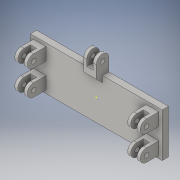
# Autodesk Inventor part: wheel mount
Saved by Autodesk Inventor 2016 (Build 200138000, 138)
## iProperties
Created: 2017-06-27
Part Number: wheel mount
Material: Generic
Document SubType Name: Modeling
Designer: andon
Density: 1 g/cm^3
Appearance: Default
Author: andon
Autodesk Inventor part; units mm, degrees
ref_plane "YZ Plane" through (0, 0, 0) normal (1, 0, 0) x (0, 1, 0)
ref_plane "XZ Plane" through (0, 0, 0) normal (0, 1, 0) x (-1, 0, 0)
ref_plane "XY Plane" through (0, 0, 0) normal (0, 0, 1) x (1, 0, 0)
sketch "Sketch1" plane through (0, 0, 0) normal (0, 0, 1) x (1, 0, 0)
  line L0 (-266.7, 88.9) -> (266.7, 88.9)
  line L1 (266.7, 88.9) -> (266.7, -88.9)
  line L2 (266.7, -88.9) -> (-266.7, -88.9)
  line L3 (-266.7, -88.9) -> (-266.7, 88.9)
  line L4 (-266.7, 88.9) -> (266.7, -88.9) construction
  line L5 (266.7, 88.9) -> (-266.7, -88.9) construction
  point P0 (0, 0)
  dimension "d0" = 533.4
  dimension "d1" = 177.8
  constraints: 12 end point, 2 midpoint, 2 parallel, 1 horizontal, 1 perpendicular
  measures "d0" distance of L1.end L2.end
  measures "d1" distance of L0.end L1.end
extrude "Extrusion1" add sketch "Sketch1" along normal blind 25.4
sketch "Sketch2" plane through (0, 0, 25.4) normal (0, 0, 1) x (1, 0, 0)
  line L0 (-254, -76.2) -> (254, -76.2)
  line L1 (254, -76.2) -> (254, 76.2)
  line L2 (254, 76.2) -> (-254, 76.2)
  line L3 (-254, 76.2) -> (-254, -76.2)
  line L4 (-254, -76.2) -> (254, 76.2) construction
  line L5 (254, -76.2) -> (-254, 76.2) construction
  line L6 (-254, 76.2) -> (-203.2, 76.2)
  line L7 (-203.2, 76.2) -> (-203.2, 25.4)
  line L8 (-203.2, 25.4) -> (-254, 25.4)
  line L9 (-254, 25.4) -> (-254, 76.2)
  line L10 (-254, -76.2) -> (-203.2, -76.2)
  line L11 (-203.2, -76.2) -> (-203.2, -25.4)
  line L12 (-203.2, -25.4) -> (-254, -25.4)
  line L13 (-254, -25.4) -> (-254, -76.2)
  line L14 (254, 76.2) -> (203.2, 76.2)
  line L15 (203.2, 76.2) -> (203.2, 25.4)
  line L16 (203.2, 25.4) -> (254, 25.4)
  line L17 (254, 25.4) -> (254, 76.2)
  line L18 (254, -76.2) -> (203.2, -76.2)
  line L19 (203.2, -76.2) -> (203.2, -25.4)
  line L20 (203.2, -25.4) -> (254, -25.4)
  line L21 (254, -25.4) -> (254, -76.2)
  point P0 (0, 0)
  dimension "d4" = 508
  dimension "d5" = 152.4
  dimension "d6" = 50.8
  dimension "d7" = 50.8
  dimension "d8" = 50.8
  dimension "d9" = 50.8
  dimension "d10" = 50.8
  dimension "d11" = 50.8
  dimension "d12" = 50.8
  dimension "d13" = 50.8
  constraints: 44 end point, 10 parallel, 5 horizontal, 5 perpendicular, 2 midpoint
  measures "d4" distance of L2.end L1.end
  measures "d5" distance of L1.end L0.end
  measures "d6" distance of L7.end L8.end
  measures "d7" distance of L6.end L7.end
  measures "d8" distance of L12.end L11.end
  measures "d9" distance of L11.end L10.end
  measures "d10" distance of L16.end L15.end
  measures "d11" distance of L15.end L14.end
  measures "d12" distance of L19.end L20.end
  measures "d13" distance of L18.end L19.end
extrude "Extrusion2" add sketch "Sketch2" along normal blind 76.2 contours L3 L12 L11 L0 | L19 L20 L1 L0 | L3 L2 L7 L8 | L16 L15 L2 L1
sketch "Sketch3" plane through (0, 0, 101.6) normal (0, 0, 1) x (1, 0, 0)
  line L0 (-254, 76.2) -> (-203.2, 76.2) projected
  line L1 (-203.2, 25.4) -> (-254, 25.4) projected
  line L2 (-241.3, 76.2) -> (-215.9, 76.2)
  line L3 (-215.9, 76.2) -> (-215.9, 25.4)
  line L4 (-215.9, 25.4) -> (-241.3, 25.4)
  line L5 (-241.3, 25.4) -> (-241.3, 76.2)
  line L6 (-254, -25.4) -> (-203.2, -25.4) projected
  line L7 (-254, -76.2) -> (-203.2, -76.2) projected
  line L8 (-241.3, -25.4) -> (-215.9, -25.4)
  line L9 (-215.9, -25.4) -> (-215.9, -76.2)
  line L10 (-215.9, -76.2) -> (-241.3, -76.2)
  line L11 (-241.3, -76.2) -> (-241.3, -25.4)
  line L12 (254, -25.4) -> (203.2, -25.4) projected
  line L13 (203.2, -76.2) -> (254, -76.2) projected
  line L14 (215.9, -25.4) -> (241.3, -25.4)
  line L15 (241.3, -25.4) -> (241.3, -76.2)
  line L16 (241.3, -76.2) -> (215.9, -76.2)
  line L17 (215.9, -76.2) -> (215.9, -25.4)
  line L18 (254, 76.2) -> (203.2, 76.2) projected
  line L19 (241.3, 25.4) -> (215.9, 25.4)
  line L20 (215.9, 25.4) -> (215.9, 76.2)
  line L21 (215.9, 76.2) -> (241.3, 76.2)
  line L22 (241.3, 76.2) -> (241.3, 25.4)
  point P0 (0, 0)
  constraints: 32 end point, 9 point on line, 8 parallel, 4 horizontal, 4 perpendicular
extrude "Extrusion3" cut sketch "Sketch3" against normal blind 50.8
fillet "Fillet1" radius 25.4 16 edges at (-247.65, 76.2, 101.6) (-209.55, 76.2, 101.6) (-209.55, 25.4, 101.6) (-247.65, 25.4, 101.6) (-247.65, -25.4, 101.6) (-247.65, -76.2, 101.6) (-209.55, -25.4, 101.6) (-209.55, -76.2, 101.6) (247.65, 76.2, 101.6) (209.55, 76.2, 101.6) (209.55, 25.4, 101.6) (247.65, 25.4, 101.6) (247.65, -25.4, 101.6) (209.55, -25.4, 101.6) (209.55, -76.2, 101.6) (247.65, -76.2, 101.6)
sketch "Sketch4" plane through (254, 25.4, 25.4) normal (1, 0, 0) x (0, 0, -1)
  arc A0 (-50.8, 50.8) -> (-50.8, 0) centre (-50.8, 25.4) ccw projected
  arc A1 (-50.8, -50.8) -> (-50.8, -101.6) centre (-50.8, -76.2) ccw projected
  circle A2 centre (-50.8, 25.4) radius 9.525
  circle A3 centre (-50.8, -76.2) radius 9.525
  point P0 (25.4, -25.4)
  dimension "d19" = 19.05
  dimension "d20" = 19.05
  constraints: 2 centre point, 2 coincident
  measures "d19" diameter of A2
  measures "d20" diameter of A3
extrude "Extrusion4" cut sketch "Sketch4" against normal blind 558.8
sketch "Sketch5" plane through (0, 0, 25.4) normal (0, 0, 1) x (1, 0, 0)
  point P0 (0, 0)
sketch "Sketch6" plane through (-266.7, 88.9, 0) normal (0, 1, 0) x (1, 0, 0)
  line L0 (0, 0) -> (533.4, 0) projected
  line L1 (0, 0) -> (533.4, 0)
  line L2 (241.3, 0) -> (292.1, 0)
  line L3 (292.1, 0) -> (292.1, -50.8)
  line L4 (292.1, -50.8) -> (241.3, -50.8)
  line L5 (241.3, -50.8) -> (241.3, 0)
  line L6 (533.4, -25.4) -> (0, -25.4) projected
  line L7 (241.3, 0) -> (292.1, -50.8) construction
  line L8 (292.1, 0) -> (241.3, -50.8) construction
  point P0 (266.7, 0)
  point P1 (266.7, -25.4)
  dimension "d23" = 50.8
  dimension "d24" = 50.8
  constraints: 14 end point, 3 equal length, 3 midpoint, 1 horizontal, 1 perpendicular
  measures "d23" distance of L3.end L4.end
  measures "d24" distance of L2.end L3.end
extrude "Extrusion5" add sketch "Sketch6" along normal blind 76.2
chamfer "Chamfer1" distance 25.4 angle 45 1 edges at (0, 88.9, 25.4)
sketch "Sketch7" plane through (-266.7, 165.1, 0) normal (0, 1, 0) x (1, 0, 0)
  line L0 (533.4, 0) -> (0, 0) projected
  line L1 (292.1, -50.8) -> (241.3, -50.8) projected
  line L2 (254, 0) -> (279.4, 0)
  line L3 (279.4, 0) -> (279.4, -50.8)
  line L4 (279.4, -50.8) -> (254, -50.8)
  line L5 (254, -50.8) -> (254, 0)
  point P0 (266.7, 0)
  constraints: 8 end point, 2 parallel, 2 point on line, 1 horizontal, 1 perpendicular
extrude "Extrusion6" cut sketch "Sketch7" against normal blind 50.8
fillet "Fillet2" radius 25.4 4 edges at (-19.05, 165.1, 50.8) (-19.05, 165.1, 0) (19.05, 165.1, 50.8) (19.05, 165.1, 0)
sketch "Sketch8" plane through (25.4, 88.9, 25.4) normal (1, 0, 0) x (0, 0, -1)
  arc A0 (25.4, 50.8) -> (-25.4, 50.8) centre (0, 50.8) ccw projected
  circle A1 centre (0, 50.8) radius 9.525
  point P0 (25.4, -88.9)
  dimension "d33" = 19.05
  constraints: 1 centre point, 1 coincident
  measures "d33" diameter of A1
extrude "Extrusion7" cut sketch "Sketch8" against normal blind 50.8
body "Solid1"
